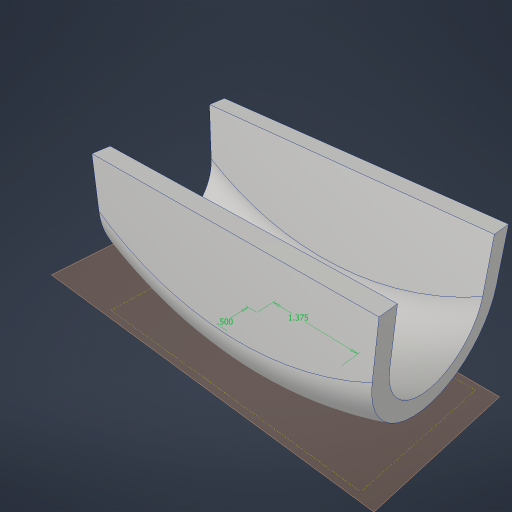
# Autodesk Inventor part: EL2-024
Saved by Autodesk Inventor 2023.4 (Build 274418000, 418)
## iProperties
Created: 2025-02-10
Part Number: EL2-024
Material: Aluminum 6061
Document SubType Name: Modeling
Designer: brand
Density: 2.7 g/cm^3
Appearance: Aluminum - Flat
Author: brand
Autodesk Inventor part; units mm, degrees
ref_plane "YZ Plane" through (0, 0, 0) normal (1, 0, 0) x (0, 1, 0)
ref_plane "XY Plane" through (0, 0, 0) normal (0, 0, 1) x (1, 0, 0)
sketch "Sketch1" plane through (0, 0, 0) normal (0, 0, 1) x (1, 0, 0)
  line L0 (-50.8, -31.75) -> (50.8, -31.75)
  line L1 (50.8, -31.75) -> (50.8, 31.75)
  line L2 (50.8, 31.75) -> (-50.8, 31.75)
  line L3 (-50.8, 31.75) -> (-50.8, -31.75)
  line L4 (-50.8, -31.75) -> (50.8, 31.75) construction
  line L5 (50.8, -31.75) -> (-50.8, 31.75) construction
  point P0 (0, 0)
  dimension "d0" = 101.6
  dimension "d1" = 63.5
  constraints: 12 end point, 2 midpoint, 2 parallel, 1 horizontal, 1 perpendicular
  measures "d0" distance of L2.end L1.end
  measures "d1" distance of L1.end L0.end
extrude "Extrusion1" add sketch "Sketch1" along normal mid plane 50.8
sketch "Sketch2" plane through (50.8, -31.75, 25.4) normal (1, 0, 0) x (0, 0, -1)
  line L0 (50.8, 63.5) -> (50.8, 0) construction
  line L1 (50.8, 0) -> (0, 0) construction
  line L2 (0, 0) -> (0, 63.5) construction
  line L3 (0, 63.5) -> (50.8, 63.5) construction
  circle A0 centre (25.4, 44.45) radius 19.05
  line L4 (50.8, 63.5) -> (0, 63.5) construction
  line L5 (6.35, 44.45) -> (44.45, 44.45)
  line L6 (44.45, 44.45) -> (44.45, 63.5)
  line L7 (44.45, 63.5) -> (6.35, 63.5)
  line L8 (6.35, 63.5) -> (6.35, 44.45)
  point P0 (25.4, 31.75)
  point P1 (44.45, 44.45)
  point P2 (25.4, 63.5)
  dimension "d4" = 38.1
  constraints: 8 end point, 2 horizontal, 2 parallel, 1 coincident, 1 midpoint, 1 perpendicular, 1 point on line, 1 vertical alignment, 3 other
sketch "Sketch3" plane through (0, 0, 0) normal (0, 0, 1) x (1, 0, 0)
  line L0 (50.8, -31.75) -> (-50.8, -31.75) construction
  line L1 (-50.8, -31.75) -> (-50.8, 31.75) construction
  line L2 (-50.8, 31.75) -> (50.8, 31.75) construction
  line L3 (50.8, 31.75) -> (50.8, -31.75) construction
  arc A0 (-50.8, 12.7) -> (50.8, 12.7) centre (0, 93.2725) ccw
  point P0 (0, 0)
  dimension "d5" = 95.25
  constraints: 2 point on circle, 1 centre point, 1 horizontal alignment, 1 point on line
  measures "d5" radius of A0
sweep "Sweep1" cut profiles "Sketch2" path "Sketch3"
extrude "Extrusion2" cut sketch "Sketch2" against normal through all contours L8 L7 A0 | A0 L5 | A0 L7 L6 picked at (29.3592, 49.4146)
sketch "Sketch5" plane through (50.8, -31.75, 25.4) normal (1, 0, 0) x (0, 0, -1)
  line L0 (50.8, 63.5) -> (50.8, 0) construction
  line L1 (50.8, 0) -> (0, 0) construction
  line L2 (0, 0) -> (0, 63.5) construction
  line L3 (0, 63.5) -> (6.35, 63.5) construction
  line L4 (6.35, 63.5) -> (6.35, 44.45) construction
  arc A0 (6.35, 44.45) -> (44.45, 44.45) centre (25.4, 44.45) ccw construction
  line L5 (44.45, 44.45) -> (44.45, 63.5) construction
  line L6 (44.45, 63.5) -> (50.8, 63.5) construction
  circle A1 centre (25.4, 44.45) radius 19.05 construction
  arc A2 (6.35, 44.45) -> (44.45, 44.45) centre (25.4, 44.45) ccw construction
  circle A3 centre (25.4, 44.45) radius 25.4
  line L7 (0, 0) -> (0, 63.5) construction
  line L8 (0, 44.45) -> (50.8, 44.45)
  line L9 (50.8, 44.45) -> (50.8, 0)
  line L10 (50.8, 0) -> (0, 0)
  line L11 (0, 0) -> (0, 44.45)
  point P0 (25.4, 31.75)
  dimension "d13" = 6.35
  constraints: 8 end point, 2 centre point, 2 parallel, 2 point on circle, 2 point on line, 1 coincident, 1 concentric, 1 horizontal, 1 perpendicular
  measures "d13" radial gap between concentric circles of A1 A3
sweep "Sweep3" cut profiles "Sketch5" path "Sketch3" contours L9 L10 L11 A3
ref_plane "Work Plane1" through (0, -24.2469, 0) normal (0, 1, 0) x (-1, 0, 0)
sketch "Sketch6" plane through (0, -24.2469, 0) normal (0, 1, 0) x (-1, 0, 0)
  line L0 (50.8, -25.4) -> (50.8, 25.4) construction
  line L1 (-50.8, -25.4) -> (50.8, -25.4) construction
  line L2 (-50.8, 25.4) -> (-50.8, -25.4) construction
  line L3 (-50.8, 25.4) -> (50.8, 25.4) construction
  line L4 (17.4625, 6.35) -> (-17.4625, 6.35)
  line L5 (-17.4625, 6.35) -> (-17.4625, -6.35)
  line L6 (-17.4625, -6.35) -> (17.4625, -6.35)
  line L7 (17.4625, -6.35) -> (17.4625, 6.35)
  line L8 (17.4625, 6.35) -> (-17.4625, -6.35) construction
  line L9 (-17.4625, 6.35) -> (17.4625, -6.35) construction
  point P0 (0, 0)
  dimension "d16" = 12.7
  dimension "d17" = 34.925
  constraints: 12 end point, 2 midpoint, 2 parallel, 1 horizontal, 1 perpendicular
  measures "d16" distance of L6.end L4.start
  measures "d17" distance of L5.end L6.end
body "Solid1"
